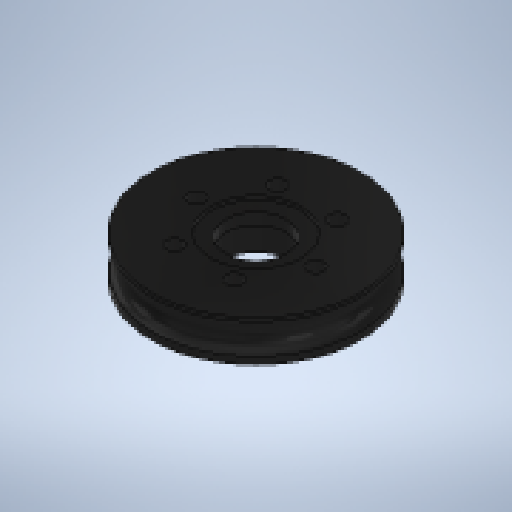
# Autodesk Inventor part: Weapon Pulley
Saved by Autodesk Inventor 2023.2 (Build 272271000, 271)
## iProperties
Created: 2023-01-09
Part Number: Weapon Pulley
Material: Nylon 6/6
Document SubType Name: Modeling
Designer: Nathan Cai
Density: 1.13 g/cm^3
Appearance: Smooth - Black
Author: Nathan Cai
Autodesk Inventor part; units mm, degrees
ref_plane "YZ Plane" through (0, 0, 0) normal (1, 0, 0) x (0, 1, 0)
ref_plane "XZ Plane" through (0, 0, 0) normal (0, 1, 0) x (-1, 0, 0)
ref_plane "XY Plane" through (0, 0, 0) normal (0, 0, 1) x (1, 0, 0)
sketch "Sketch1" plane through (0, 0, 0) normal (0, 1, 0) x (-1, 0, 0)
  circle A0 centre (0, 0) radius 7.1437
  circle A1 centre (0, 0) radius 22.225
  line L0 (0, 0) -> (0, -38.1) construction
  circle A2 centre (0, -38.1) radius 15.875 construction
  dimension "d0" = 14.2875
  dimension "PulleyOD_W" = 44.45
  dimension "d2" = 38.1
  dimension "PulleyOD_M" = 31.75
  constraints: 3 centre point, 3 coincident, 2 end point, 1 tangent, 1 vertical
  measures "d0" diameter of A0
  measures "PulleyOD_W" diameter of A1
  measures "d2" distance of L0.start L0.end
  measures "PulleyOD_M" diameter of A2
extrude "Extrusion1" add sketch "Sketch1" along normal blind 8.7312
sketch "Sketch2" plane through (0, 0, 0) normal (1, 0, 0) x (0, 1, 0)
  line L0 (8.7312, -22.225) -> (8.7312, 22.225) projected
  line L1 (8.7312, 0) -> (0, 0) construction
  line L2 (0, -22.225) -> (8.7312, -22.225) projected
  circle A0 centre (4.7625, -22.225) radius 3.175
  dimension "d12" = 6.35
  dimension "d13" = 3.9688
  constraints: 2 end point, 1 centre point, 1 horizontal, 1 midpoint, 1 point on line
  measures "d12" diameter of A0
  measures "d13" distance from line of L0 A0.centre
revolve "Revolution1" cut sketch "Sketch2" angle 360 about axis through (0, 8.7312, 0) along (0, -1, 0)
sketch "Sketch3" plane through (0, 8.7312, 0) normal (0, 1, 0) x (1, 0, 0)
  circle A0 centre (0, 0) radius 9.525
  dimension "d14" = 19.05
  constraints: 1 centre point, 1 coincident
  measures "d14" diameter of A0
extrude "Extrusion2" cut sketch "Sketch3" against normal blind 0.7937
sketch "Sketch4" plane through (0, 7.9375, 0) normal (0, 1, 0) x (1, 0, 0)
  circle A0 centre (0, 0) radius 7.1437
  circle A1 centre (0, 0) radius 7.1437 projected
  circle A2 centre (0, 0) radius 6.35
  dimension "d17" = 14.2875
  dimension "d18" = 12.7
  constraints: 2 centre point, 2 coincident
  measures "d17" diameter of A0
  measures "d18" diameter of A2
extrude "Extrusion3" add sketch "Sketch4" against normal blind 2.3813
sketch "Sketch5" plane through (0, 8.7312, 0) normal (0, 1, 0) x (1, 0, 0)
  circle A0 centre (0, 0) radius 12.7 construction
  line L0 (0, 0) -> (12.7, 0) construction
  circle A1 centre (12.7, 0) radius 1.7526
  circle A2 centre (0, 0) radius 15.875 construction
  circle A3 centre (0, 0) radius 22.225 projected
  circle A4 centre (0, 0) radius 12.7 construction
  circle A5 centre (6.35, 10.9985) radius 1.7526
  circle A6 centre (-6.35, 10.9985) radius 1.7526
  circle A7 centre (-12.7, 0) radius 1.7526
  circle A8 centre (-6.35, -10.9985) radius 1.7526
  circle A9 centre (6.35, -10.9985) radius 1.7526
  dimension "d21" = 25.4
  dimension "d23" = 3.5052
  dimension "d28" = 6.35
  dimension "d29" = 3.175
  dimension "d40" = 360
  constraints: 8 centre point, 3 coincident, 2 end point, 1 horizontal, 1 horizontal alignment, 15 other
  measures "d23" diameter of A1
  measures "d28" radial gap between concentric circles of A3 A2
  measures "d29" radial gap between concentric circles of A2 A4
extrude "Extrusion4" cut sketch "Sketch5" against normal through all contours A1 | A5 | A6 | A7 | A8 | A9
equation "\"d2\" = Pulley_Spacing"
equation "\"Pulley_Spacing\" = 38.1"
body "Solid1"
